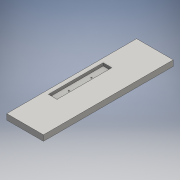
# Autodesk Inventor part: Part18
Saved by Autodesk Inventor 2016 (Build 200138000, 138)
## iProperties
Created: 2016-03-16
Part Number: Part18
Material: Generic
Document SubType Name: Modeling
Designer: sims01
Density: 1 g/cm^3
Appearance: Default
Author: sims01
Autodesk Inventor part; units mm, degrees
ref_plane "YZ Plane" through (0, 0, 0) normal (1, 0, 0) x (0, 1, 0)
ref_plane "XZ Plane" through (0, 0, 0) normal (0, 1, 0) x (-1, 0, 0)
ref_plane "XY Plane" through (0, 0, 0) normal (0, 0, 1) x (1, 0, 0)
sketch "Sketch1" plane through (0, 0, 0) normal (0, 0, 1) x (1, 0, 0)
  line L0 (-30, 230) -> (100, 230)
  line L1 (100, 230) -> (100, -230)
  line L2 (100, -230) -> (-30, -230)
  line L3 (-30, -230) -> (-30, 230)
  point P0 (0, 0)
  dimension "d0" = 30
  dimension "d1" = 100
  dimension "d2" = 460
  dimension "d3" = 230
  constraints: 8 end point, 2 parallel, 1 horizontal, 1 perpendicular
  measures "d0" distance from line of L3 point (0, 0)
  measures "d1" distance from line of L1 point (0, 0)
  measures "d2" distance of L2.end L0.start
  measures "d3" distance from line of point (0, 0) L2
extrude "baseExtrusion" add sketch "Sketch1" along normal blind 10
sketch "Sketch2" plane through (0, 0, 10) normal (0, 0, 1) x (1, 0, 0)
  line L0 (-30, 230) -> (-30, -230) projected
  point P0 (0, 0)
  point P1 (0, 40)
  point P2 (0, -40)
  dimension "d6" = 80
  dimension "d7" = 40
  dimension "d8" = 30
  dimension "d9" = 30
  constraints: 1 vertical alignment
  measures "d6" distance of point (0, -40) point (0, 40)
  measures "d7" distance of point (0, 0) point (0, 40)
  measures "d8" distance from line of point (0, 40) L0
  measures "d9" distance from line of point (0, 0) L0
hole "xyStageAttatchM5" at (0, 40, 10) at (0, -40, 10) direction (0, 0, -1) diameter 4.134 depth 14.2 tip angle 118 thread size "M5x0.8" class "6H" standard "ISO Metric profile"
sketch "Sketch3" plane through (0, 0, 10) normal (0, 0, 1) x (1, 0, 0)
  line L0 (-30, 230) -> (100, 230)
  line L1 (100, 230) -> (100, -230)
  line L2 (100, -230) -> (-30, -230)
  line L3 (-30, -230) -> (-30, 230)
  line L4 (100, 230) -> (-30, 230) projected
  line L5 (-30, -230) -> (100, -230) projected
  line L6 (100, -230) -> (100, 230) projected
  line L7 (-30, 230) -> (-30, -230) projected
  line L8 (-15.3915, 97.0335) -> (15.3915, 97.0335)
  line L9 (15.3915, 97.0335) -> (15.3915, -97.0335)
  line L10 (15.3915, -97.0335) -> (-15.3915, -97.0335)
  line L11 (-15.3915, -97.0335) -> (-15.3915, 97.0335)
  point P0 (0, 0)
  dimension "d17" = 194.0669
  dimension "d18" = 97.0335
  dimension "d19" = 30.783
  dimension "d20" = 15.3915
  constraints: 16 end point, 4 collinear, 4 parallel, 2 horizontal, 2 perpendicular
  measures "d17" distance of L8.end L9.end
  measures "d18" distance from line of point (0, 0) L8
  measures "d19" distance between parallel lines of L9 L11
  measures "d20" distance from line of point (0, 0) L9
extrude "Extrusion2" add sketch "Sketch3" along normal blind 10
equation "\"d3\" = 0.5 * d2"
equation "\"d7\" = 0.5 * d6"
equation "\"d8\" = d9"
equation "\"d18\" = 0.5 * d17"
equation "\"d20\" = 0.5 * d19"
body "Solid1"
